Autodesk Inventor part; units mm, degrees
(part 3 of 3)
  line L414 (51.25, -11.75) -> (40.75, -11.75)
  line L415 (40.75, -11.75) -> (40.75, -1.25)
  line L416 (40.75, -1.25) -> (51.25, -1.25)
  line L417 (51.25, -1.25) -> (51.25, -11.75)
  line L418 (51.25, 3.25) -> (40.75, 3.25)
  line L419 (40.75, 3.25) -> (40.75, 13.75)
  line L420 (40.75, 13.75) -> (51.25, 13.75)
  line L421 (51.25, 13.75) -> (51.25, 3.25)
  line L422 (51.25, 18.25) -> (40.75, 18.25)
  line L423 (40.75, 18.25) -> (40.75, 28.75)
  line L424 (40.75, 28.75) -> (51.25, 28.75)
  line L425 (51.25, 28.75) -> (51.25, 18.25)
  line L426 (51.25, 33.25) -> (40.75, 33.25)
  line L427 (40.75, 33.25) -> (40.75, 43.75)
  line L428 (40.75, 43.75) -> (51.25, 43.75)
  line L429 (51.25, 43.75) -> (51.25, 33.25)
  line L430 (51.25, 48.25) -> (40.75, 48.25)
  line L431 (40.75, 48.25) -> (40.75, 58.75)
  line L432 (40.75, 58.75) -> (51.25, 58.75)
  line L433 (51.25, 58.75) -> (51.25, 48.25)
  line L434 (51.25, 63.25) -> (40.75, 63.25)
  line L435 (40.75, 63.25) -> (40.75, 73.75)
  line L436 (40.75, 73.75) -> (51.25, 73.75)
  line L437 (51.25, 73.75) -> (51.25, 63.25)
  line L438 (51.25, 78.25) -> (40.75, 78.25)
  line L439 (40.75, 78.25) -> (40.75, 88.75)
  line L440 (40.75, 88.75) -> (51.25, 88.75)
  line L441 (51.25, 88.75) -> (51.25, 78.25)
  line L442 (51.25, 93.25) -> (40.75, 93.25)
  line L443 (40.75, 93.25) -> (40.75, 103.75)
  line L444 (40.75, 103.75) -> (51.25, 103.75)
  line L445 (51.25, 103.75) -> (51.25, 93.25)
  line L446 (51.25, 108.25) -> (40.75, 108.25)
  line L447 (40.75, 108.25) -> (40.75, 118.75)
  line L448 (40.75, 118.75) -> (51.25, 118.75)
  line L449 (51.25, 118.75) -> (51.25, 108.25)
  line L450 (10.75, -86.75) -> (21.25, -86.75)
  line L451 (21.25, -86.75) -> (21.25, -68.75)
  line L452 (21.25, -68.75) -> (10.75, -68.75)
  line L453 (10.75, -68.75) -> (10.75, -86.75)
  line L454 (10.75, -64.25) -> (21.25, -64.25)
  line L455 (21.25, -64.25) -> (21.25, -53.75)
  line L456 (21.25, -53.75) -> (10.75, -53.75)
  line L457 (10.75, -53.75) -> (10.75, -64.25)
  line L458 (11.75, -64.5) -> (20.25, -64.5) projected
  line L459 (10.75, -31.25) -> (21.25, -31.25)
  line L460 (21.25, -31.25) -> (21.25, -49.25)
  line L461 (21.25, -49.25) -> (10.75, -49.25)
  line L462 (10.75, -49.25) -> (10.75, -31.25)
  line L463 (10.75, -26.75) -> (21.25, -26.75)
  line L464 (21.25, -26.75) -> (21.25, -8.75)
  line L465 (21.25, -8.75) -> (10.75, -8.75)
  line L466 (10.75, -8.75) -> (10.75, -26.75)
  line L467 (10.75, 13.75) -> (21.25, 13.75)
  line L468 (21.25, 13.75) -> (21.25, -4.25)
  line L469 (21.25, -4.25) -> (10.75, -4.25)
  line L470 (10.75, -4.25) -> (10.75, 13.75)
  line L471 (10.75, 18.25) -> (21.25, 18.25)
  line L472 (21.25, 18.25) -> (21.25, 36.25)
  line L473 (21.25, 36.25) -> (10.75, 36.25)
  line L474 (10.75, 36.25) -> (10.75, 18.25)
  line L475 (10.75, 40.75) -> (21.25, 40.75)
  line L476 (21.25, 40.75) -> (21.25, 51.25)
  line L477 (21.25, 51.25) -> (10.75, 51.25)
  line L478 (10.75, 51.25) -> (10.75, 40.75)
  line L479 (11.75, 40.5) -> (20.25, 40.5) projected
  line L480 (10.75, 73.75) -> (21.25, 73.75)
  line L481 (21.25, 73.75) -> (21.25, 55.75)
  line L482 (21.25, 55.75) -> (10.75, 55.75)
  line L483 (10.75, 55.75) -> (10.75, 73.75)
  line L484 (10.75, 78.25) -> (21.25, 78.25)
  line L485 (21.25, 78.25) -> (21.25, 96.25)
  line L486 (21.25, 96.25) -> (10.75, 96.25)
  line L487 (10.75, 96.25) -> (10.75, 78.25)
  line L488 (10.75, 118.75) -> (21.25, 118.75)
  line L489 (21.25, 118.75) -> (21.25, 100.75)
  line L490 (21.25, 100.75) -> (10.75, 100.75)
  line L491 (10.75, 100.75) -> (10.75, 118.75)
  point P0 (0, 0)
  dimension "d223" = 0.25
  dimension "d224" = 10.5
  dimension "d225" = 10.5
  dimension "d226" = 0.25
  dimension "d229" = 15
  dimension "d232" = 15
  dimension "d235" = 18
  dimension "d236" = 10.5
  dimension "d237" = 0.25
  dimension "d238" = 18
  dimension "d239" = 18
  dimension "d240" = 18
  dimension "d241" = 18
  dimension "d242" = 10.5
  dimension "d243" = 0.25
  dimension "d244" = 18
  dimension "d245" = 18
  dimension "d246" = 18
  constraints: 976 end point, 22 parallel, 12 horizontal, 12 point on line, 11 perpendicular, 2 collinear, 1 vertical, 886 other
  measures "d223" distance between parallel lines of L4 L0
  measures "d224" distance of L0.start L0.end
  measures "d225" distance of L0.end L1.end
  measures "d226" distance between parallel lines of L5 L3
  measures "d229" distance of L0.start L6.start
  measures "d232" distance of L0.start L66.start
  measures "d235" distance of L450.end L451.end
  measures "d236" distance of L454.end L455.end
  measures "d237" distance between parallel lines of L458 L454
  measures "d238" distance of L459.end L460.end
  measures "d239" distance of L465.end L282.end
  measures "d240" distance of L467.end L468.end
  measures "d241" distance of L473.end L294.end
  measures "d242" distance of L475.end L476.end
  measures "d243" distance between parallel lines of L479 L475
  measures "d244" distance of L480.end L481.end
  measures "d245" distance of L484.end L485.end
  measures "d246" distance of L488.end L489.end
extrude "Extrusion8" add sketch "Sketch21" along normal blind 1 contours L0 L1 L2 L3 | L6 L7 L8 L9 | L66 L67 L68 L69 | L70 L71 L72 L73 | L130 L131 L132 L133 | L134 L135 L136 L137 | L162 L163 L164 L165 | L166 L167 L168 L169 | L170 L171 L172 L173 | L174 L175 L176 L177 | L178 L179 L180 L181 | L182 L183 L184 L185 | L186 L187 L188 L189 | L190 L191 L192 L193 | L194 L195 L196 L197 | L198 L199 L200 L201 | L226 L227 L228 L229 | L230 L231 L232 L233 | L234 L235 L236 L237 | L238 L239 L240 L241 | L242 L243 L244 L245 | L246 L247 L248 L249 | L250 L251 L252 L253 | L254 L255 L256 L257 | L258 L259 L260 L261 | L262 L263 L264 L265 | L266 L267 L268 L269 | L268 L453 L270 L451 | L270 L271 L452 L273 | L454 L271 L272 L273 | L272 L457 L274 L455 | L274 L275 L456 L277 | L461 L275 L276 L277 | L276 L462 L278 L460 | L278 L279 L280 L281 | L282 L283 L284 L285 | L284 L466 L286 L464 | L286 L287 L465 L289 | L469 L287 L288 L289 | L288 L470 L290 L468 | L290 L291 L292 L293 | L294 L295 L296 L297 | L296 L474 L298 L472 | L298 L299 L473 L301 | L475 L299 L300 L301 | L300 L478 L302 L476 | L302 L303 L477 L305 | L482 L303 L304 L305 | L304 L483 L306 L481 | L306 L307 L308 L309 | L310 L311 L312 L313 | L312 L487 L314 L485 | L314 L315 L486 L317 | L490 L315 L316 L317 | L316 L491 L318 L489 | L318 L319 L320 L321 | L322 L323 L324 L325 | L326 L327 L328 L329 | L330 L331 L332 L333 | L334 L335 L336 L337 | L338 L339 L340 L341 | L342 L343 L344 L345 | L346 L347 L348 L349 | L350 L351 L352 L353 | L354 L355 L356 L357 | L358 L359 L360 L361 | L362 L363 L364 L365 | L366 L367 L368 L369 | L370 L371 L372 L373 | L374 L375 L376 L377 | L378 L379 L380 L381 | L382 L383 L384 L385 | L386 L387 L388 L389 | L390 L391 L392 L393 | L394 L395 L396 L397 | L398 L399 L400 L401 | L402 L403 L404 L405 | L406 L407 L408 L409 | L410 L411 L412 L413 | L414 L415 L416 L417 | L418 L419 L420 L421 | L422 L423 L424 L425 | L426 L427 L428 L429 | L430 L431 L432 L433 | L434 L435 L436 L437 | L438 L439 L440 L441 | L442 L443 L444 L445 | L446 L447 L448 L449
body "Solid1"
